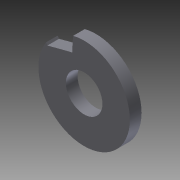
# Autodesk Inventor part: Gear Washer Spacer
Saved by Autodesk Inventor 2014 SP1 (Build 180222100, 222)
## iProperties
Created: 2012-03-30
Part Number: Gear Washer Spacer
Material: Steel
Document SubType Name: Modeling
Designer: Moses
Mass: 2.51195 g
Surface Area: 4.60053 cm^2
Volume: 0.319994 cm^3
Density: 7.85 g/cm^3
Appearance: Steel
Author: Moses
Autodesk Inventor part; units mm, degrees
ref_plane "YZ Plane" through (0, 0, 0) normal (1, 0, 0) x (0, 1, 0)
ref_plane "XZ Plane" through (0, 0, 0) normal (0, 1, 0) x (-1, 0, 0)
ref_plane "XY Plane" through (0, 0, 0) normal (0, 0, 1) x (1, 0, 0)
sketch "Sketch1" plane through (0, 0, 0) normal (0, 0, 1) x (1, 0, 0)
  circle A0 centre (0, 0) radius 7.9375
  circle A1 centre (0, 0) radius 3.175
  dimension "d0" = 15.875
  dimension "d1" = 6.35
  constraints: 2 centre point, 2 coincident
  measures "d0" diameter of A0
  measures "d1" diameter of A1
extrude "Extrusion1" add sketch "Sketch1" along normal blind 2.032
sketch "Sketch2" plane through (0, 0, 0) normal (0, 0, -1) x (-1, 0, 0)
  arc A0 (5.4488, 5.2173) -> (0.9937, 5.4324) centre (-5.2691, -170.5112) ccw projected
  arc A1 (0.9937, 5.4324) -> (-3.3435, 17.439) centre (-61.406, -10.3219) ccw projected
  arc A2 (10.9226, 16.7501) -> (5.4488, 5.2173) centre (66.0404, -16.4757) ccw projected
  arc A3 (5.5974, 5.6279) -> (0.309, 7.9315) centre (0, 0) ccw
  circle A4 centre (0, 0) radius 7.9375 construction
  dimension "d4" = 7.9375
  constraints: 6 point on circle, 1 centre point
  measures "d4" radius of A3
extrude "Extrusion2" cut sketch "Sketch2" against normal blind 25.4
body "Solid1"
